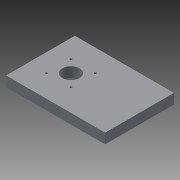
# Autodesk Inventor part: CNC-Z-axis- top plate
Saved by Autodesk Inventor 2015 (Build 190159000, 159)
## iProperties
Created: 2015-03-21
Part Number: CNC-Z-axis- top plate
Material: Generic
Document SubType Name: Modeling
Designer: Bangladesh
Density: 1 g/cm^3
Appearance: Default
Author: Bangladesh
Autodesk Inventor part; units mm, degrees
ref_plane "YZ Plane" through (0, 0, 0) normal (1, 0, 0) x (0, 1, 0)
ref_plane "XZ Plane" through (0, 0, 0) normal (0, 1, 0) x (-1, 0, 0)
ref_plane "XY Plane" through (0, 0, 0) normal (0, 0, 1) x (1, 0, 0)
sketch "Sketch1" plane through (0, 0, 0) normal (0, 1, 0) x (-1, 0, 0)
  line L0 (63.994, 44.45) -> (-63.994, 44.45)
  line L1 (-63.994, 44.45) -> (-63.994, -44.45)
  line L2 (-63.994, -44.45) -> (63.994, -44.45)
  line L3 (63.994, -44.45) -> (63.994, 44.45)
  line L4 (63.994, 44.45) -> (-63.994, -44.45) construction
  line L5 (-63.994, 44.45) -> (63.994, -44.45) construction
  point P0 (0, 0)
  dimension "d0" = 127.988
  dimension "d1" = 88.9
  constraints: 12 end point, 2 midpoint, 2 parallel, 1 horizontal, 1 perpendicular
  measures "d0" distance of L1.end L2.end
  measures "d1" distance of L0.end L1.end
extrude "Extrusion1" add sketch "Sketch1" along normal mid plane 13
sketch "Sketch4" plane through (0, 6.5, 0) normal (0, 1, 0) x (1, 0, 0)
  line L0 (-45.781, -21.125) -> (-3.531, -21.125)
  line L1 (-3.531, -21.125) -> (-3.531, 21.125)
  line L2 (-3.531, 21.125) -> (-45.781, 21.125)
  line L3 (-45.781, 21.125) -> (-45.781, -21.125)
  line L4 (-45.781, -21.125) -> (-3.531, 21.125) construction
  line L5 (-3.531, -21.125) -> (-45.781, 21.125) construction
  line L6 (-63.994, 44.45) -> (-63.994, -44.45) projected
  line L7 (-40.416, -15.76) -> (-8.896, -15.76)
  line L8 (-8.896, -15.76) -> (-8.896, 15.76)
  line L9 (-8.896, 15.76) -> (-40.416, 15.76)
  line L10 (-40.416, 15.76) -> (-40.416, -15.76)
  line L11 (-40.416, -15.76) -> (-8.896, 15.76) construction
  line L12 (-8.896, -15.76) -> (-40.416, 15.76) construction
  circle A0 centre (-40.416, -15.76) radius 1.3891
  circle A1 centre (-40.416, 15.76) radius 1.3891
  circle A2 centre (-8.896, -15.76) radius 1.3891
  circle A3 centre (-8.896, 15.76) radius 1.3891
  circle A4 centre (-24.656, 0) radius 11
  dimension "d33" = 42.25
  dimension "d34" = 42.25
  dimension "d35" = 18.213
  dimension "d36" = 31.52
  dimension "d37" = 31.52
  dimension "d38" = 2.7781
  dimension "d39" = 2.7781
  dimension "d40" = 2.7781
  dimension "d41" = 2.7781
  dimension "d42" = 22
  constraints: 24 end point, 6 midpoint, 5 centre point, 4 coincident, 4 parallel, 2 horizontal, 2 perpendicular
  measures "d33" distance of L2.end L1.end
  measures "d34" distance of L0.end L1.end
  measures "d35" distance between parallel lines of L6 L3
  measures "d36" distance of L9.end L8.end
  measures "d37" distance of L8.end L7.end
  measures "d38" diameter of A0
  measures "d39" diameter of A1
  measures "d40" diameter of A2
  measures "d41" diameter of A3
  measures "d42" diameter of A4
extrude "Extrusion2" cut sketch "Sketch4" against normal blind 25.4 contours L10 A0 L7 | L7 A0 L10 | A2 L8 L7 | L7 L8 A2 | A1 L9 L10 | L10 L9 A1 | A3 L9 L8 | L8 L9 A3 | A4
body "Solid1"
